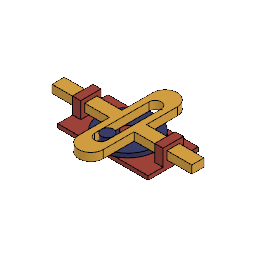
Scotch-yoke v3 (Autodesk Fusion 360 design; units mm, degrees)
Autodesk Fusion 360 part; units mm, degrees
sketch "Base" plane through (0, 0, 0) normal (0, 0, 1) x (1, 0, 0)
  line L0 (110, 61.1111) -> (-110, 61.1111)
  line L1 (-110, 61.1111) -> (-110, -61.1111)
  line L2 (-110, -61.1111) -> (110, -61.1111)
  line L3 (110, -61.1111) -> (110, 61.1111)
  line L4 (110, 61.1111) -> (-110, -61.1111) construction
  line L5 (-110, 61.1111) -> (110, -61.1111) construction
  circle A0 centre (0, 0) radius 10
  dimension "d1" = 20
  dimension "d18" = 20
  dimension "d65" = 220
  constraint horizontal L0
  constraint perpendicular L0 L1
  constraint parallel L0 L2
  constraint parallel L1 L3
  constraint coincident L4 A0.centre
  constraint coincident L5 A0.centre
  constraint coincident A0.centre origin
  measures "d1" diameter of A0
  measures "d18" diameter of A0
  measures "d65" distance of L0.start L0.end
extrude "Extrude1" add sketch "Base" along normal blind 10 makes body 1
extrude "Extrude2" add sketch "Base" along normal blind 20 contours A0 bodies 1
sketch "Support right" plane through (0, 0, 0) normal (1, 0, 0) x (0, 1, 0)
  line L0 (-25, 10, 100) -> (25, 10, 100)
  line L1 (25, 10, 100) -> (25, 50, 100)
  line L2 (25, 50, 100) -> (-25, 50, 100)
  line L3 (-25, 50, 100) -> (-25, 10, 100)
  line L4 (-15, 20, 100) -> (15, 20, 100)
  line L5 (15, 20, 100) -> (15, 40, 100)
  line L6 (15, 40, 100) -> (-15, 40, 100)
  line L7 (-15, 40, 100) -> (-15, 20, 100)
extrude "Extrude3" add sketch "Support right" along normal mid plane 20 contours L0 L1 L2 L3 in plane through (100, 0, 0) normal (1, 0, 0) bodies 1
sketch "Support left" plane through (0, 0, 0) normal (1, 0, 0) x (0, 1, 0)
  line L0 (25, 10, -100) -> (-25, 10, -100)
  line L1 (-25, 10, -100) -> (-25, 50, -100)
  line L2 (-25, 50, -100) -> (25, 50, -100)
  line L3 (25, 50, -100) -> (25, 10, -100)
  line L4 (15, 19.8649, -100) -> (-15, 19.8649, -100)
  line L5 (-15, 19.8649, -100) -> (-15, 40, -100)
  line L6 (-15, 40, -100) -> (15, 40, -100)
  line L7 (15, 40, -100) -> (15, 19.8649, -100)
  dimension "d15" = 9.8649
extrude "Extrude4" add sketch "Support left" along normal mid plane 20 contours L0 L1 L2 L3 in plane through (-100, 0, 0) normal (1, 0, 0) bodies 1
sketch "Crank" plane through (0, 0, 10) normal (0, 0, 1) x (-1, 0, 0)
  circle A0 centre (0, 0) radius 10
  line L0 (110, -25) -> (90, -25)
  line L1 (90, -25) -> (90, 25)
  line L2 (90, 25) -> (110, 25)
  line L3 (110, 25) -> (110, 61.1111)
  line L4 (110, 61.1111) -> (-110, 61.1111)
  line L5 (-110, 61.1111) -> (-110, 25)
  line L6 (-110, 25) -> (-90, 25)
  line L7 (-90, 25) -> (-90, -25)
  line L8 (-90, -25) -> (-110, -25)
  line L9 (-110, -25) -> (-110, -61.1111)
  line L10 (-110, -61.1111) -> (110, -61.1111)
  line L11 (110, -61.1111) -> (110, -25)
  circle A1 centre (0, 0) radius 67.8694
  circle A2 centre (0, 0) radius 15
  dimension "d25" = 30
  constraint concentric A0 A1
  constraint concentric A1 A2
  measures "d25" diameter of A2
move_face "OffsetFaces1" offset 4.7 1 faces at (9.9503, -0.9957, 13.3333) on bodies 1
extrude "Extrude7" add sketch "Crank" along normal blind 10 separate body contours L10 A1 | L4 L10 A1 | L4 A1 makes body 2
extrude "Extrude8" add 1 faces at (4.1033, 3.4906, 20) along direction (0, 0, 1) blind 30 on bodies 1 bodies 1
sketch "Conection part" plane through (0, 0, 20) normal (0, 0, 1) x (-1, 0, 0)
  circle A0 centre (0, 0) radius 15
  circle A1 centre (0, 0) radius 67.8694
  line L0 (15, 0) -> (-15, 0)
  line L1 (15, 0) -> (-15, 0)
  line L2 (15, -66.1911) -> (15, 0)
  line L3 (-15, 0) -> (-15, 66.1911)
  line L4 (15, 66.1911) -> (15, 0)
  arc A2 (-15, -65.8439) -> (15, -65.8439) centre (0, -65.8439) ccw
  arc A3 (15, 65.8439) -> (-15, 65.8439) centre (0, 65.8439) ccw
  line L5 (-15, 15) -> (-15, -15)
  line L6 (-15, -15) -> (-80, -15)
  line L7 (-80, -15) -> (-170, -15)
  line L8 (-170, 15) -> (-170, -15)
  line L9 (0, -80.8439) -> (0, 80.8439)
  line L10 (15, -15) -> (80, -15)
  line L11 (80, -15) -> (170, -15)
  line L12 (80, 15) -> (170, 15)
  line L13 (80, 15) -> (15, 15)
  line L14 (170, 15) -> (170, -15)
  line L15 (-170, 15) -> (-15, 15)
  line L16 (-30, 90) -> (-30, -90)
  line L17 (30, -90) -> (30, 90)
  arc A4 (30, 90) -> (-30, 90) centre (0, 90) ccw
  arc A5 (-15, -64.0192) -> (-17.4404, -65.5903) centre (0, -90) ccw
  arc A6 (-30, -90) -> (30, -90) centre (0, -90) ccw
  line L18 (-15, 0) -> (-15, -64.0192)
  line L19 (-15, -65.8439) -> (-15, -66.1911)
  point P0 (-100, 15)
  dimension "d31" = 30
  dimension "d32" = 30
  dimension "d33" = 65
  constraint coincident A0 L0.start
  constraint coincident A0 L0.end
  constraint horizontal L0
  constraint horizontal L1
  constraint vertical L18
  constraint vertical L2
  constraint symmetric L0.start L1 L2.end
  constraint symmetric L0.end L1 L3.start
  constraint symmetric L1 A2 A3
  constraint coincident A1 L2.start
  constraint coincident A1 L19.end
  constraint coincident L2 A2.end
  constraint coincident A2.start L18
  constraint coincident A1 L4.start
  constraint coincident A1 L3.end
  constraint coincident L3 A3.end
  constraint coincident L4 A3.start
  constraint vertical L5
  constraint horizontal L6
  constraint coincident L5.end L18
  constraint perpendicular L7 L8
  constraint midpoint A2 L9.start
  constraint midpoint A3 L9.end
  constraint vertical L9
  constraint symmetric L5.start L9 L13.end
  constraint symmetric L5.end L9 L10.start
  constraint symmetric L6.end L9 L10.end
  constraint symmetric L7.end L9 L11.end
  constraint symmetric L8.start L9 L12.end
  constraint perpendicular L3 L15
  constraint vertical L16
  constraint vertical L17
  constraint coincident A1 A5.end
  constraint concentric A5 A6
  constraint collinear L18 L19
  measures "d31" distance of L0.start L0.end
  measures "d32" diameter of A2
  measures "d33" distance of L5.end L6.end
extrude "Extrude9" add sketch "Conection part" along normal blind 19.7 separate body contours L2 L4 L10 L13 L17 | A1 L2 L10 L17 | A1 L4 L13 L17 | L3 L5 L6 L15 L16 L18 | A1 L10 L13 L17 | A1 L3 L15 L16 | A1 L6 L16 A5 L18 | A1 A3 L16 L17 A4 | A1 A2 L16 L17 A6 | A1 L10 L11 L12 L13 L14 | A1 L6 L15 L16 | A1 L6 L7 L8 L15 makes body 3
copy_body "Body->Comp1" bodies 1 removing the originals makes body 4 in component "Base"
copy_body "Body->Comp2" bodies 2 removing the originals makes body 5 in component "Crank"
copy_body "Body->Comp3" bodies 3 removing the originals makes body 6 in component "Conection part"
sketch "Sketch8" plane through (0, 0, 20) normal (0, 0, 1) x (-1, 0, 0)
  circle A0 centre (0, 0) radius 15
  circle A1 centre (0, 0) radius 67.8694
  circle A2 centre (0, 50) radius 15
  dimension "d53" = 30
  measures "d53" diameter of A2
extrude "Extrude1'" add sketch "Sketch8" along normal blind 20 contours A2 bodies 5 in component "Crank"
move_face "OffsetFaces1'" offset -30 1 faces at (4.1033, 3.4906, 50) on bodies 4 in component "Base"
component "Base" placed x (1, 0, 0) y (0, 1, 0) z (0, 0, 1) at (0, 0, 0)
component "Crank" placed x (1, 0, 0) y (0, 1, 0) z (0, 0, 1) at (0, 0, 0)
component "Conection part" placed x (1, 0, 0) y (0, 1, 0) z (0, 0, 1) at (0, 0, 0)
named bodies: "Base", "Crank", "Conection part"
